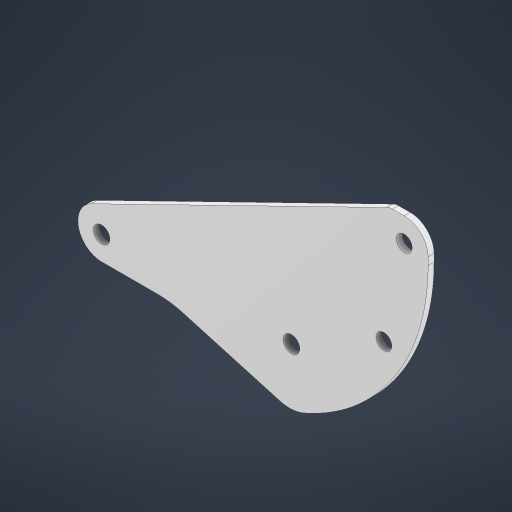
# Autodesk Inventor part: sled_front
Saved by Autodesk Inventor 2024 (Build 280153000, 153)
## iProperties
Created: 2023-08-16
Part Number: sled_front
Material: Acetal Resin, White
Document SubType Name: Sheet Metal
Designer: avere
Density: 1.425 g/cm^3
Appearance: Smooth - White
Flat Pattern Width: 4.30261 cm
Flat Pattern Length: 10.2313 cm
Flat Pattern Area: 44.0214 cm^2
Sheet Metal Rule: Default_mm
Sheet Metal Width: 1.694 in
Sheet Metal Length: 4.028 in
Sheet Metal Area: 6.823 in^2
Author: avere
Autodesk Inventor part; units mm, degrees
ref_plane "YZ Plane" through (0, 0, 0) normal (1, 0, 0) x (0, 1, 0)
ref_plane "XZ Plane" through (0, 0, 0) normal (0, 1, 0) x (-1, 0, 0)
ref_plane "XY Plane" through (0, 0, 0) normal (0, 0, 1) x (1, 0, 0)
sketch "Sketch1" plane through (0, 0, 0) normal (0, 0, 1) x (1, 0, 0)
  circle A0 centre (32.4279, -12.9523) radius 2.1844
  line L0 (68.9404, 23.5133) -> (68.9404, 25.4755)
  line L1 (62.5658, 31.8255) -> (59.4204, 31.8133)
  arc A1 (68.9404, 25.4755) -> (62.5658, 31.8255) centre (62.5904, 25.4755) ccw
  line L2 (-3.5614, -19.3023) -> (-18.3721, -19.3023)
  arc A2 (35.7428, -27.2531) -> (68.9404, 23.5133) centre (13.525, 23.5133) ccw
  line L3 (29.3044, -27.6849) -> (3.4241, -20.2818)
  arc A3 (29.3044, -27.6849) -> (35.7428, -27.2531) centre (31.9239, -18.5272) ccw
  arc A4 (3.4241, -20.2818) -> (-3.5614, -19.3023) centre (-3.5614, -44.7023) ccw
  circle A5 centre (62.5904, 25.4755) radius 2.0955
  arc A6 (59.4204, 31.8133) -> (57.8679, 31.4009) centre (59.4327, 28.6383) ccw
  circle A7 centre (-18.3721, -12.9523) radius 2.1844
  arc A8 (-21.1618, -7.2479) -> (-18.3721, -19.3023) centre (-18.3721, -12.9523) ccw
  line L4 (-21.1618, -7.2479) -> (57.8679, 31.4009)
  point P0 (0, 0)
  point P1 (-20.4601, 31.5039)
  point P2 (32.4279, -28.5784)
  point P3 (58.5866, 31.8101)
  dimension "d4" = 6.35
  dimension "d21" = 9.525
  dimension "d22" = 25.4
  dimension "d24" = 4.191
  dimension "d28" = 3.175
  dimension "d30" = 4.3688
  constraints: 13 point on circle, 10 end point, 9 centre point, 9 tangent, 3 point on line, 2 coincident, 2 vertical, 1 other
  measures "d4" radius of A1
  measures "d21" radius of A3
  measures "d22" radius of A4
  measures "d24" diameter of A5
  measures "d28" radius of A6
  measures "d30" diameter of A7
extrude "Extrusion1" add sketch "Sketch1" along normal blind 1.5875
sketch "Sketch2" plane through (0, 0, 1.5875) normal (0, 0, 1) x (1, 0, 0)
  circle A0 centre (57.15, 0) radius 2.0828
  point P0 (0, 0)
  dimension "d7" = 4.1656
  constraints: 1 centre point
  measures "d7" diameter of A0
extrude "Extrusion2" cut sketch "Sketch2" against normal blind 1.5875
equation "\"BendRadius\" = Thickness"
equation "\"BendReliefWidth\" = Thickness"
equation "\"BendReliefDepth\" = 0.5 * Thickness"
equation "\"CornerReliefSize\" = 4 * Thickness"
equation "\"MinimumRemnant\" = 2 * Thickness"
equation "\"TransitionRadius\" = BendRadius"
equation "\"JacobiRadiusSize\" = BendRadius"
equation "\"GapSize\" = Thickness"
equation "\"Thickness\" = 1.5875"
body "Solid1"
